MarsRoverMeasures (Autodesk Fusion 360 design; units mm, degrees)
Autodesk Fusion 360 part; units mm, degrees
mesh "Mesh1" [no effect]
ref_plane "WorkPlane2" through (0, 0, 68) normal (0, 0, 1) x (1, 0, 0)
sketch "Top - Wheel" plane through (0, 0, 68) normal (0, 0, 1) x (1, 0, 0)
  line L0 (-376.5767, 66.1614) -> (-266.5767, 66.1614)
  line L1 (-266.5767, 66.1614) -> (-266.5767, -58.8386)
  line L2 (-266.5767, -58.8386) -> (-376.5767, -58.8386)
  line L3 (-376.5767, -58.8386) -> (-376.5767, 66.1614)
  line L4 (293.4233, -58.8386) -> (293.4233, 66.1614)
  line L5 (293.4233, 66.1614) -> (403.4233, 66.1614)
  line L6 (403.4233, 66.1614) -> (403.4233, -58.8386)
  line L7 (403.4233, -58.8386) -> (293.4233, -58.8386)
  line L8 (-376.5767, 3.6614) -> (403.4233, 3.6614) construction
  line L9 (-341.5767, 366.1614) -> (-231.5767, 366.1614)
  line L10 (-231.5767, 366.1614) -> (-231.5767, 241.1614)
  line L11 (-231.5767, 241.1614) -> (-341.5767, 241.1614)
  line L12 (-341.5767, 241.1614) -> (-341.5767, 366.1614)
  line L13 (-341.5767, -393.8386) -> (-341.5767, -268.8386)
  line L14 (-341.5767, -268.8386) -> (-231.5767, -268.8386)
  line L15 (-231.5767, -268.8386) -> (-231.5767, -393.8386)
  line L16 (-231.5767, -393.8386) -> (-341.5767, -393.8386)
  line L17 (258.4233, 241.1614) -> (258.4233, 366.1614)
  line L18 (258.4233, 366.1614) -> (368.4233, 366.1614)
  line L19 (368.4233, 366.1614) -> (368.4233, 241.1614)
  line L20 (368.4233, 241.1614) -> (258.4233, 241.1614)
  line L21 (258.4233, -393.8386) -> (258.4233, -268.8386)
  line L22 (258.4233, -268.8386) -> (368.4233, -268.8386)
  line L23 (368.4233, -393.8386) -> (258.4233, -393.8386)
  line L24 (368.4233, -268.8386) -> (368.4233, -393.8386)
  line L25 (-341.5767, 303.6614) -> (368.4233, 303.6614) construction
  line L26 (-341.5767, -331.3386) -> (368.4233, -331.3386) construction
  line L27 (-266.5767, 66.1614) -> (-266.5767, -58.8386) construction
  line L28 (-231.5767, 241.1614) -> (-231.5767, -268.8386) construction
  line L29 (-321.5767, 66.1614) -> (-321.5767, -58.8386) construction
  line L30 (348.4233, 66.1614) -> (348.4233, -58.8386) construction
  line L31 (-286.5767, 366.1614) -> (-286.5767, 241.1614) construction
  line L32 (313.4233, 366.1614) -> (313.4233, 241.1614) construction
  dimension "d3" = 125
  dimension "d4" = 110
  dimension "d9" = 125
  dimension "d10" = 110
  dimension "d11" = 125
  dimension "d12" = 110
  dimension "d13" = 125
  dimension "d14" = 110
  dimension "d15" = 125
  dimension "d16" = 110
  dimension "d17" = 125
  dimension "d18" = 110
  dimension "d20" = 35
  dimension "d21" = 670
  dimension "d22" = 600
  dimension "d25" = 300
  dimension "d26" = 335
  dimension "d27" = 490
  dimension "d28" = 560
  dimension "d29" = 760
  dimension "d30" = 710
  dimension "d31" = 780
  dimension "d212" = 780
  constraint horizontal L0
  constraint vertical L1
  constraint horizontal L2
  constraint vertical L3
  constraint horizontal L5
  constraint vertical L6
  constraint horizontal L7
  constraint vertical L4
  constraint midpoint L3 L8.start
  constraint midpoint L6 L8.end
  constraint perpendicular L6 L8
  constraint horizontal L9
  constraint vertical L10
  constraint horizontal L11
  constraint vertical L12
  constraint horizontal L14
  constraint vertical L15
  constraint horizontal L16
  constraint vertical L13
  constraint horizontal L18
  constraint vertical L19
  constraint horizontal L20
  constraint vertical L17
  constraint horizontal L22
  constraint vertical L24
  constraint horizontal L23
  constraint vertical L21
  constraint midpoint L12 L25.start
  constraint midpoint L19 L25.end
  constraint perpendicular L19 L25
  constraint midpoint L13 L26.start
  constraint midpoint L24 L26.end
  constraint perpendicular L24 L26
  constraint perpendicular L14 L27
  constraint perpendicular L14 L28
  constraint midpoint L0 L29.start
  constraint perpendicular L2 L29
  constraint midpoint L5 L30.start
  constraint perpendicular L7 L30
  constraint midpoint L9 L31.start
  constraint perpendicular L11 L31
  constraint midpoint L18 L32.start
  constraint perpendicular L20 L32
  constraint midpoint L2 L29.end
  constraint midpoint L7 L30.end
  constraint midpoint L11 L31.end
  constraint midpoint L20 L32.end
  measures "d3" distance of L0.start L2.end
  measures "d4" distance of L0.start L0.end
  measures "d9" distance of L4.start L4.end
  measures "d10" distance of L5.end L4.end
  measures "d11" distance of L9.start L11.end
  measures "d12" distance of L9.start L9.end
  measures "d13" distance of L13.start L13.end
  measures "d14" distance of L14.end L13.end
  measures "d15" distance of L17.start L17.end
  measures "d16" distance of L18.end L17.end
  measures "d17" distance of L21.end L21.start
  measures "d18" distance of L22.end L21.end
  measures "d20" distance of L1.end L28
  measures "d21" distance of L29 L30
  measures "d22" distance of L31 L32
  measures "d25" vertical distance of L8.end L25.end
  measures "d26" vertical distance of L8.end L26.end
  measures "d27" distance of L10.end L17.start
  measures "d28" distance of L1.end L4.start
  measures "d29" distance of L18.end L23.start
  measures "d30" distance of L9.start L18.end
  measures "d31" distance of L0.start L5.end
  measures "d212" distance of L0.start L5.end
ref_plane "WorkPlane3" through (-300, 0, 0) normal (1, 0, 0) x (0, 1, 0)
sketch "Left - Wheel and suspension" plane through (-300, 0, 0) normal (1, 0, 0) x (0, 1, 0)
  line L0 (303.5438, 69.637) -> (-331.4562, 69.637) construction
  circle A0 centre (303.5438, 69.637) radius 62.5
  circle A1 centre (-331.4562, 69.637) radius 62.5
  circle A2 centre (3.5438, 69.637) radius 62.5
  line L1 (-82.4562, 251.637) -> (130.5438, 182.8899)
  line L2 (303.5438, 69.637) -> (303.5438, 201.4155)
  line L3 (303.5438, 201.4155) -> (130.5438, 182.8899)
  line L4 (3.5438, 69.637) -> (3.5438, 107.637)
  line L5 (3.5438, 107.637) -> (130.5438, 182.8899)
  line L6 (-331.4562, 69.637) -> (-331.4562, 193.637)
  line L7 (-331.4562, 193.637) -> (-82.4562, 251.637)
  line L8 (-167.471, 243.4821) -> (-216.657, 232.0251) construction
  line L9 (-213.4962, 209.1456) -> (-162.2533, 221.0817) construction
  line L10 (-167.471, 243.4821) -> (-162.2533, 221.0817) construction
  line L11 (72.0716, 138.0036) -> (92.522, 150.1213) construction
  line L12 (83.8559, 164.7466) -> (59.0651, 150.057) construction
  line L13 (83.8559, 164.7466) -> (92.522, 150.1213) construction
  dimension "d33" = 635
  dimension "d34" = 125
  dimension "d35" = 125
  dimension "d36" = 125
  dimension "d37" = 300
  dimension "d38" = 335
  dimension "d58" = 149
  dimension "d59" = 156
  dimension "d60" = 124
  dimension "d62" = 182
  dimension "d63" = 249
  dimension "d64" = 213
  dimension "d65" = 173
  dimension "d66" = 134.8386
  dimension "d67" = 113.2529
  dimension "d68" = 38
  dimension "d69" = 120.649
  dimension "d70" = 147.6212
  dimension "d71" = 170.1624
  dimension "d400" = 23
  dimension "d401" = 17
  dimension "d454" = 155.464
  dimension "d475" = 103.112
  constraint horizontal L0
  constraint coincident L0.start A0.centre
  constraint coincident L0.end A1.centre
  constraint coincident L0 A2.centre
  constraint perpendicular L0 L2
  constraint coincident A2.centre L4.start
  constraint perpendicular L0 L4
  constraint perpendicular L0 L6
  constraint parallel L7 L9
  constraint perpendicular L9 L10
  constraint perpendicular L8 L10
  constraint parallel L5 L11
  constraint perpendicular L11 L13
  constraint perpendicular L12 L13
  measures "d33" distance of L0.start L0.end
  measures "d34" diameter of A0
  measures "d35" diameter of A1
  measures "d36" diameter of A2
  measures "d37" distance of L0.start A2.centre
  measures "d38" distance of L0.end A2.centre
  measures "d58" angle of L1 L7
  measures "d59" angle of L1 L3
  measures "d60" distance of L0.end L6.end
  measures "d62" vertical distance of L0.end L1.start
  measures "d63" horizontal distance of L1.start L6.end
  measures "d64" horizontal distance of L1.start L1.end
  measures "d65" horizontal distance of L1.end L2.end
  measures "d67" distance of L0 L1.end
  measures "d68" distance of A2.centre L4.end
  measures "d69" angle of L4 L5
  measures "d70" distance of L1.end L4.end
  measures "d71" distance of L1.end A2.centre
  measures "d400" distance of L8.start L9.end
  measures "d401" distance of L11.end L12.start
  measures "d454" angle of L3 L5
  measures "d475" angle of L6 L7
sketch "Left - RTG" plane through (0, 0, 0) normal (1, 0, 0) x (0, 1, 0)
  line L0 (0, 0) -> (0, 467.5219) construction
  line L1 (0, 277.6823) -> (561.1829, 277.6823) construction
  line L2 (210.2843, 277.6823) -> (472.4121, 429.0222) construction
  dimension "d476" = 30
  constraint coincident L0.start origin
  constraint vertical L0
  constraint coincident L0 L1.start
  constraint perpendicular L0 L1
  constraint coincident L1 L2.start
  measures "d476" angle of L1 L2
ref_plane "WorkPlane22" through (12.125, 0, 0) normal (0, 0.866025, 0.5) x (1, 0, 0)
ref_plane "WorkPlane23" through (12.125, 313.5012, 181) normal (0, 0.866025, 0.5) x (1, 0, 0)
ref_plane "WorkPlane4" through (0, 0, 178) normal (0, 0, 1) x (1, 0, 0)
sketch "Top - Wheel and suspension" plane through (0, 0, 178) normal (0, 0, 1) x (1, 0, 0)
  line L0 (-285.6566, 303.5772) -> (-285.6566, -331.4228) construction
  line L1 (-285.6566, 3.5772) -> (-371.3267, 3.5772) construction
  line L2 (-266.7956, 128.5772) -> (-194.7956, 128.5772) construction
  line L3 (-285.6566, 303.5772) -> (-245.2546, 128.5772) construction
  line L4 (-245.2546, 128.5772) -> (-245.2546, -8.4343) construction
  line L5 (-285.6566, -331.4228) -> (-209.2546, -103.3688) construction
  line L6 (-209.2546, -103.3688) -> (-209.2546, 128.5772) construction
  line L7 (-225.0074, -83.4228) -> (-155.0074, -83.4228) construction
  line L8 (-148.5074, 179.005) -> (174.4926, 179.005)
  line L9 (174.4926, 179.005) -> (174.4926, -256.995)
  line L10 (174.4926, -256.995) -> (-148.5074, -256.995)
  line L11 (-148.5074, -256.995) -> (-148.5074, 179.005)
  line L12 (-266.2546, 66.0772) -> (-376.2546, 66.0772)
  line L13 (-376.2546, 66.0772) -> (-376.2546, -58.9228)
  line L14 (-376.2546, -58.9228) -> (-266.2546, -58.9228)
  line L15 (-266.2546, -58.9228) -> (-266.2546, 66.0772)
  line L16 (-199.9544, -33.4769) -> (-199.9544, 51.6617) construction
  line L17 (-221.947, -32.9072) -> (-221.947, 52.0545) construction
  dimension "d73" = 635
  dimension "d74" = 300
  dimension "d75" = 335
  dimension "d76" = 72
  dimension "d77" = 175
  dimension "d78" = 125
  dimension "d79" = 167
  dimension "d80" = 161.478
  dimension "d81" = 70
  dimension "d82" = 87
  dimension "d83" = 248
  dimension "d84" = 436
  dimension "d85" = 323
  dimension "d86" = 6.5
  dimension "d87" = 36
  dimension "d88" = 110
  dimension "d89" = 125
  dimension "d90" = 62.5
  dimension "d91" = 21
  dimension "d211" = 22
  dimension "d473" = 18.522
  dimension "d474" = 13
  constraint vertical L0
  constraint coincident L0 L1.start
  constraint perpendicular L0 L1
  constraint horizontal L2
  constraint coincident L2 L3.end
  constraint perpendicular L2 L4
  constraint coincident L2 L6.end
  constraint perpendicular L2 L6
  constraint perpendicular L6 L7
  constraint horizontal L8
  constraint vertical L9
  constraint horizontal L10
  constraint vertical L11
  constraint horizontal L12
  constraint vertical L13
  constraint horizontal L14
  constraint vertical L15
  constraint perpendicular L2 L16
  constraint vertical L17
  measures "d73" distance of L0.start L0.end
  measures "d74" distance of L0.start L1
  measures "d75" distance of L0.end L1.start
  measures "d76" distance of L2.start L2.end
  measures "d77" vertical distance of L0.start L2.start
  measures "d78" vertical distance of L1.start L2.start
  measures "d79" angle of L3 L4
  measures "d80" angle of L5 L6
  measures "d81" distance of L7.start L7.end
  measures "d82" vertical distance of L1.start L7.start
  measures "d83" vertical distance of L0.end L7.start
  measures "d84" distance of L8.end L9.end
  measures "d85" distance of L9.end L10.end
  measures "d86" distance of L7.end L11
  measures "d87" distance of L3.end L6.end
  measures "d88" distance of L12.start L12.end
  measures "d89" distance of L12.start L14.end
  measures "d90" distance of L1.end L14
  measures "d91" distance of L4.end L15
  measures "d211" distance of L16.start L17.start
  measures "d473" angle of L0 L5
  measures "d474" angle of L0 L3
sketch "Top - Chassis" plane through (0, 0, 178) normal (0, 0, 1) x (1, 0, 0)
  line L0 (311.1042, 304.5371) -> (-284.8958, 304.5371) construction
  line L1 (-284.8958, 304.5371) -> (-284.8958, -330.4629) construction
  line L2 (-284.8958, -330.4629) -> (311.1042, -330.4629) construction
  line L3 (311.1042, -330.4629) -> (311.1042, 304.5371) construction
  line L4 (-266.8958, 64.6219) -> (-376.8958, 64.6219)
  line L5 (-376.8958, 64.6219) -> (-376.8958, -60.3781)
  line L6 (-376.8958, -60.3781) -> (-266.8958, -60.3781)
  line L7 (-266.8958, -60.3781) -> (-266.8958, 64.6219)
  line L8 (403.1042, -60.3781) -> (403.1042, 64.6219)
  line L9 (403.1042, 64.6219) -> (293.1042, 64.6219)
  line L10 (293.1042, 64.6219) -> (293.1042, -60.3781)
  line L11 (293.1042, -60.3781) -> (403.1042, -60.3781)
  line L12 (174.6042, 178.5371) -> (-148.3958, 178.5371)
  line L13 (-148.3958, 178.5371) -> (-148.3958, -256.4629)
  line L14 (-148.3958, -256.4629) -> (174.6042, -256.4629)
  line L15 (174.6042, -256.4629) -> (174.6042, 178.5371)
  line L16 (-341.6412, 372.3911) -> (368.3588, 372.3911) construction
  line L17 (-341.6412, -397.6089) -> (368.3588, -397.6089) construction
  line L18 (-341.6412, 372.3911) -> (-341.6412, -397.6089) construction
  line L19 (368.3588, 372.3911) -> (368.3588, -397.6089) construction
  line L20 (174.6042, -38.9629) -> (-148.3958, -38.9629) construction
  line L21 (174.6042, 17.0371) -> (-148.3958, 17.0371) construction
  line L22 (-148.3958, -87.6567) -> (-165.872, -87.6567)
  dimension "d93" = 635
  dimension "d94" = 596
  dimension "d95" = 110
  dimension "d96" = 125
  dimension "d97" = 110
  dimension "d98" = 125
  dimension "d99" = 18
  dimension "d100" = 18
  dimension "d101" = 780
  dimension "d102" = 323
  dimension "d103" = 435
  dimension "d106" = 136.5
  dimension "d107" = 136.5
  dimension "d109" = 126
  dimension "d110" = 74
  dimension "d241" = 710
  dimension "d402" = 770
  dimension "d455" = 56
  constraint horizontal L0
  constraint vertical L1
  constraint horizontal L2
  constraint vertical L3
  constraint horizontal L4
  constraint vertical L5
  constraint horizontal L6
  constraint vertical L7
  constraint horizontal L9
  constraint vertical L10
  constraint horizontal L11
  constraint vertical L8
  constraint horizontal L12
  constraint vertical L13
  constraint horizontal L14
  constraint vertical L15
  constraint horizontal L17
  constraint coincident L17 L18.end
  constraint coincident L17 L19.end
  constraint midpoint L15 L20.start
  constraint midpoint L13 L20.end
  constraint coincident L15 L21.start
  constraint coincident L13 L21.end
  constraint perpendicular L13 L21
  constraint coincident L13 L22.start
  constraint perpendicular L13 L22
  measures "d93" distance of L0.start L2.end
  measures "d94" distance of L0.start L0.end
  measures "d95" distance of L4.start L4.end
  measures "d96" distance of L4.start L6.end
  measures "d97" distance of L9.end L8.end
  measures "d98" distance of L8.start L8.end
  measures "d99" distance of L1 L6.end
  measures "d100" distance of L3 L10.end
  measures "d101" distance of L4.end L8.end
  measures "d102" distance of L12.start L12.end
  measures "d103" distance of L12.start L14.end
  measures "d106" horizontal distance of L2.end L14.end
  measures "d107" horizontal distance of L1.end L13.end
  measures "d109" vertical distance of L0.start L12.start
  measures "d110" vertical distance of L2.end L14.end
  measures "d241" distance of L16.start L16.end
  measures "d402" distance of L16.start L17.start
  measures "d455" distance of L20 L21
ref_plane "WorkPlane5" through (0, -225, 0) normal (0, 1, 0) x (0, 0, 1)
sketch "Front - Chassis and Cam" plane through (0, -225, 0) normal (0, 1, 0) x (1, 0, 0)
  line L0 (-148.2843, -313) -> (174.7157, -313)
  line L1 (174.7157, -313) -> (174.7157, -185)
  line L2 (174.7157, -185) -> (-148.2843, -185)
  line L3 (-148.2843, -185) -> (-148.2843, -313)
  line L4 (-53.8892, -564) -> (-202.3892, -564)
  line L5 (-202.3892, -564) -> (-202.3892, -571)
  line L6 (-202.3892, -571) -> (-53.8892, -571)
  line L7 (-53.8892, -571) -> (-53.8892, -564)
  line L8 (-196.9099, -614) -> (-70.9099, -614)
  line L9 (-70.9099, -614) -> (-70.9099, -571)
  line L10 (-70.9099, -571) -> (-196.9099, -571)
  line L11 (-196.9099, -571) -> (-196.9099, -614)
  line L12 (-189.3792, -621) -> (-77.8792, -621)
  line L13 (-70.9099, -571) -> (-60.6099, -571)
  line L14 (-60.6099, -571) -> (-60.6099, -585.7)
  line L15 (-60.6099, -585.7) -> (-70.9099, -585.7)
  line L16 (-70.9099, -585.7) -> (-70.9099, -571)
  line L17 (-158.5751, -506.4898) -> (-128.2751, -506.4898)
  line L18 (-128.2751, -506.4898) -> (-128.2751, -485.8898)
  line L19 (-128.2751, -485.8898) -> (-158.5751, -485.8898)
  line L20 (-158.5751, -485.8898) -> (-158.5751, -506.4898)
  dimension "d112" = 323
  dimension "d113" = 128
  dimension "d114" = 148.5
  dimension "d115" = 7
  dimension "d116" = 43
  dimension "d117" = 126
  dimension "d118" = 111.5
  dimension "d119" = 7
  dimension "d120" = 251
  dimension "d124" = 14.7
  dimension "d125" = 10.3
  dimension "d213" = 30.3
  dimension "d215" = 20.6
  dimension "d388" = 571
  constraint horizontal L0
  constraint vertical L1
  constraint horizontal L2
  constraint vertical L3
  constraint horizontal L4
  constraint vertical L5
  constraint horizontal L6
  constraint vertical L7
  constraint horizontal L8
  constraint vertical L9
  constraint horizontal L10
  constraint vertical L11
  constraint coincident L6 L9.end
  constraint horizontal L12
  constraint horizontal L13
  constraint vertical L14
  constraint horizontal L15
  constraint vertical L16
  constraint horizontal L17
  constraint vertical L18
  constraint horizontal L19
  constraint vertical L20
  measures "d112" distance of L0.start L0.end
  measures "d113" distance of L0.end L1.end
  measures "d114" distance of L5 L7
  measures "d115" distance of L4.end L5.end
  measures "d116" distance of L8.start L10.end
  measures "d117" distance of L8.start L8.end
  measures "d118" distance of L12.start L12.end
  measures "d119" vertical distance of L8.end L12.end
  measures "d120" distance of L0.start L4
  measures "d124" distance of L13.end L14.end
  measures "d125" distance of L14.end L15.end
  measures "d213" distance of L18.end L19.end
  measures "d215" distance of L17.start L19.end
  measures "d388" vertical distance of origin L9.end
ref_plane "WorkPlane10" through (-386.1613, -337.5, 781.806) normal (0, 0, 1) x (1, 0, 0)
sketch "Sketch19" plane through (0, 0, 781.806) normal (0, 0, 1) x (-1, 0, 0)
  circle A0 centre (142.453, 225.0109) radius 33
  circle A1 centre (143.6218, 222.8237) radius 15
  dimension "d392" = 30
  measures "d392" diameter of A1
ref_plane "WorkPlane11" through (0, -220, 0) normal (0, 1, 0) x (0, 0, 1)
sketch "Sketch20" plane through (0, -220, 0) normal (0, 1, 0) x (1, 0, 0)
  line L0 (-158.6064, -506.0999) -> (-128.6064, -506.0999)
  line L1 (-128.6064, -506.0999) -> (-128.6064, -486.0999)
  line L2 (-128.6064, -486.0999) -> (-158.6064, -486.0999)
  line L3 (-158.6064, -486.0999) -> (-158.6064, -506.0999)
  line L4 (-128.6064, -486.0999) -> (-158.6064, -486.0999)
  line L5 (-200.2466, -474.0999) -> (-113.4124, -474.0999) construction
  line L6 (-201.8884, -563.5999) -> (-61.2389, -563.5999) construction
  line L7 (-181.6393, -535.0999) -> (-87.5081, -535.0999) construction
  dimension "d394" = 20
  dimension "d395" = 30
  dimension "d396" = 12
  dimension "d397" = 28.5
  dimension "d398" = 29
  dimension "d399" = 89.7
  constraint horizontal L0
  constraint vertical L1
  constraint horizontal L2
  constraint vertical L3
  constraint horizontal L4
  constraint horizontal L5
  constraint horizontal L6
  constraint parallel L6 L7
  measures "d394" distance of L0.start L2.end
  measures "d395" distance of L0.start L0.end
  measures "d396" distance of L2 L5
  measures "d397" distance of L6 L7
  measures "d398" distance of L0 L7
extrude "Extrude20" add sketch "Sketch19" along normal blind 21 contours A1
ref_plane "WorkPlane12" through (0, -260, 0) normal (0, 1, 0) x (0, 0, 1)
sketch "Sketch21" plane through (0, -260, 0) normal (0, 1, 0) x (1, 0, 0)
  circle A0 centre (-190.1986, -557.4012) radius 4.5
  line L0 (-183.1986, -551.9012) -> (-197.1986, -551.9012)
  line L1 (-197.1986, -551.9012) -> (-197.1986, -562.9012)
  line L2 (-197.1986, -562.9012) -> (-183.1986, -562.9012)
  line L3 (-183.1986, -562.9012) -> (-183.1986, -551.9012)
  line L4 (-183.1986, -551.9012) -> (-197.1986, -562.9012) construction
  line L5 (-197.1986, -551.9012) -> (-183.1986, -562.9012) construction
  point P0 (-190.1986, -557.4012)
  dimension "d403" = 9
  dimension "d405" = 11
  dimension "d406" = 14
  constraint perpendicular L0 L1
  constraint parallel L0 L2
  constraint parallel L1 L3
  constraint horizontal L0
  constraint coincident L4 P0
  constraint coincident L5 P0
  constraint coincident P0 A0.centre
  measures "d403" diameter of A0
  measures "d405" distance of L0.start L2.end
  measures "d406" distance of L0.start L0.end
sketch "Sketch24" plane through (0, 0, 310.1429) normal (0, 0, 1) x (-1, 0, 0)
  line L0 (154.6751, 110.682) -> (148.6751, 121.682)
  line L1 (148.6751, 121.682) -> (147.6751, 121.682)
  line L2 (147.6751, 121.682) -> (147.6751, 55.682)
  line L3 (147.6751, 55.682) -> (154.6751, 55.682)
  line L4 (154.6751, 55.682) -> (154.6751, 110.682)
ref_plane "WorkPlane13" through (0, 0, 250) normal (0, 0, 1) x (1, 0, 0)
sketch "Sketch25" plane through (0, 0, 250) normal (0, 0, 1) x (1, 0, 0)
ref_plane "WorkPlane14" through (192.3249, -83.182, 249.1429) normal (1, 0, 0) x (0, -1, 0)
sketch "Sketch27" plane through (192.3249, -83.182, 249.1429) normal (1, 0, 0) x (0, 1, 0)
  line L0 (88.1106, 71.7156) -> (-35.2917, 71.7156) construction
  circle A0 centre (0.3753, -3.4844) radius 19.5
  line L1 (0.3753, -3.4844) -> (0.3753, 71.7156) construction
  line L2 (-19.1247, -3.4844) -> (19.8753, -3.4844) construction
  line L3 (-3.4747, 71.7156) -> (-17.6247, -3.4844)
  circle A1 centre (0.3753, -3.4844) radius 18
  circle A2 centre (0.3753, 71.7156) radius 3.85
  dimension "d418" = 39
  dimension "d420" = 36
  dimension "d421" = 7.7
  dimension "d422" = 75.2
  constraint horizontal L0
  constraint coincident A0.centre L1.start
  constraint coincident L0 L1.end
  constraint perpendicular L0 L1
  constraint coincident A0 L2.start
  constraint coincident A0 L2.end
  constraint coincident A0.centre L2
  constraint horizontal L2
  constraint coincident L2 L3.end
  constraint coincident L3.end A1
  constraint coincident L0 L3.start
  constraint coincident L1.end A2.centre
  constraint coincident L3.start A2
  measures "d418" diameter of A0
  measures "d420" diameter of A1
  measures "d421" diameter of A2
  measures "d422" distance of A0.centre L1.end
sketch "Sketch28" plane through (0, 0, 250) normal (0, 0, 1) x (1, 0, 0)
sketch "Sketch29" plane through (0, 0, 250) normal (0, 0, 1) x (1, 0, 0)
sketch "Sketch30" plane through (0, 0, 250) normal (0, 0, 1) x (1, 0, 0)
ref_plane "WorkPlane15" through (0, -80, 0) normal (0, 1, 0) x (0, 0, 1)
sketch "Sketch31" plane through (0, -80, 0) normal (0, 1, 0) x (1, 0, 0)
  line L0 (-218.1313, -260.6757) -> (-224.4446, -230.974)
  line L1 (-214.1751, -224.3429) -> (-214.1751, -267.3429)
  line L2 (-219.1751, -265.3429) -> (-219.1751, -226.3429)
  line L3 (-219.1751, -245.8429) -> (-221.288, -245.8429)
  line L4 (-221.288, -245.8429) -> (-221.288, -245.8249)
  line L5 (-221.288, -245.8249) -> (-219.1751, -245.8249)
  line L6 (-219.1751, -245.8249) -> (-219.1751, -245.8429)
  line L7 (-216.1751, -260.2599) -> (-222.4883, -230.5582)
  line L8 (-219.1751, -260.5202) -> (-219.1751, -230)
  line L9 (-219.1751, -245.8429) -> (-219.1751, -260.3429)
  line L10 (-219.1751, -245.8429) -> (-219.1751, -231.3429)
  line L11 (-249.7499, -267.3964) -> (-256.0631, -237.6947)
  dimension "d424" = 2
  dimension "d427" = 12
  dimension "d428" = 14.5
  dimension "d429" = 14.5
  dimension "d430" = 3
  dimension "d431" = -32.3249
  constraint horizontal L3
  constraint vertical L4
  constraint horizontal L5
  constraint vertical L6
  constraint midpoint L0 L4.end
  constraint midpoint L2 L3.start
  constraint coincident L2 L8.start
  constraint perpendicular L3 L8
  constraint perpendicular L5 L9
  constraint perpendicular L5 L10
  measures "d427" angle of L7 L8
  measures "d428" distance of L3.start L9.end
  measures "d429" distance of L3.start L10.end
  measures "d430" distance of L7.start L8
ref_plane "WorkPlane16" through (-239.4269, -82.182, 248.833) normal (0.198827, -0.292372, 0.935407) x (-0.978148, 0, 0.207912)
sketch "Sketch32" plane through (-210.6129, -80.4381, 243.2534) normal (0.198827, -0.292372, 0.935407) x (-0.978148, 0, 0.207912)
  line L0 (39.7719, 116.5078) -> (31.2227, 82.2187)
  line L1 (17.4551, 122.072) -> (8.9059, 87.7829)
  line L2 (5, 0) -> (26.9699, 0)
  line L3 (18.6443, 21.3232) -> (-8.8557, 21.3232)
  line L4 (-8.8557, 21.3232) -> (-8.8557, -17.5495)
  line L5 (-8.8557, -17.5495) -> (18.6443, -17.5495)
  line L6 (18.6443, -17.5495) -> (18.6443, 21.3232)
  dimension "d433" = 23
  dimension "d435" = 76
  dimension "d436" = 27.5
  dimension "d437" = 14
  constraint horizontal L2
  constraint horizontal L3
  constraint vertical L4
  constraint horizontal L5
  constraint vertical L6
  measures "d435" angle of L0 L2
  measures "d436" distance of L3.start L3.end
  measures "d437" angle of L1 L4
ref_plane "WorkPlane17" through (0, 0, 320) normal (0, 0, 1) x (1, 0, 0)
sketch "Sketch33" plane through (0, 0, 320) normal (0, 0, 1) x (1, 0, 0)
  line L0 (-167.1178, 16.9441) -> (191.8822, 16.9441) construction
  circle A0 centre (-167.1178, 16.9441) radius 3
  circle A1 centre (191.8822, 16.9441) radius 3
  circle A2 centre (12.3822, 16.9441) radius 12.5
  circle A3 centre (12.3822, 16.9441) radius 18.5
  circle A4 centre (-167.1178, 16.9441) radius 6.25
  circle A5 centre (191.8822, 16.9441) radius 6.25
  line L1 (12.3822, 36.9441) -> (12.3822, -3.0559) construction
  line L2 (-9.2181, -3.0559) -> (33.9826, -3.0559)
  line L3 (-20.1178, 36.9441) -> (44.8822, 36.9441)
  line L4 (-20.1178, 36.9441) -> (-167.6987, 23.167)
  line L5 (-9.2181, -3.0559) -> (-167.6591, 10.7176)
  line L6 (33.9826, -3.0559) -> (192.4235, 10.7176)
  line L7 (44.8822, 36.9441) -> (192.4631, 23.167)
  dimension "d439" = 359
  dimension "d440" = 6
  dimension "d441" = 6
  dimension "d442" = 25
  dimension "d443" = 37
  dimension "d444" = 12.5
  dimension "d445" = 12.5
  dimension "d446" = 20
  dimension "d447" = 65
  dimension "d448" = 20
  constraint horizontal L0
  constraint coincident L0.start A0.centre
  constraint coincident L0.end A1.centre
  constraint midpoint L0 A2.centre
  constraint concentric A2 A3
  constraint concentric A0 A4
  constraint concentric A1 A5
  constraint perpendicular L0 L1
  constraint perpendicular L1 L3
  constraint midpoint L1.start L3
  constraint midpoint L1.end L2
  constraint horizontal L2
  constraint midpoint A2.centre L1
  constraint coincident A4 L4.end
  constraint tangent A4 L4
  constraint coincident A4 L5.end
  constraint tangent A4 L5
  constraint coincident A5 L6.end
  constraint tangent A5 L6
  constraint coincident A5 L7.end
  constraint tangent A5 L7
  measures "d439" distance of L0.start L0.end
  measures "d440" diameter of A0
  measures "d441" diameter of A1
  measures "d442" diameter of A2
  measures "d443" diameter of A3
  measures "d444" diameter of A4
  measures "d445" diameter of A5
  measures "d446" distance of A2.centre L1.end
  measures "d447" distance of L3.start L3.end
  measures "d448" vertical distance of A2.centre L1.start
ref_plane "WorkPlane18" through (0, 0, 180) normal (0, 0, 1) x (1, 0, 0)
sketch "Sketch34" plane through (0, 0, 180) normal (0, 0, 1) x (1, 0, 0)
  line L0 (-227.4262, 140.0762) -> (-260.9262, 140.0762)
  line L1 (-260.9262, 140.0762) -> (-260.9262, 117.0762)
  line L2 (-260.9262, 117.0762) -> (-227.4262, 117.0762)
  line L3 (-227.4262, 117.0762) -> (-227.4262, 140.0762)
  line L4 (-194.9262, 145.571) -> (-227.4262, 145.571)
  line L5 (-227.4262, 145.571) -> (-227.4262, 112.071)
  line L6 (-227.4262, 112.071) -> (-194.9262, 112.071)
  line L7 (-194.9262, 112.071) -> (-194.9262, 145.571)
  dimension "d450" = 33.5
  dimension "d451" = 32.5
  dimension "d452" = 23
  dimension "d453" = 33.5
  constraint horizontal L0
  constraint vertical L1
  constraint horizontal L2
  constraint vertical L3
  constraint horizontal L4
  constraint vertical L5
  constraint horizontal L6
  constraint vertical L7
  constraint coincident L2.end L5
  measures "d450" distance of L4.start L6.end
  measures "d451" distance of L4.start L4.end
  measures "d452" distance of L0.start L2.end
  measures "d453" distance of L1.end L2.end
ref_plane "WorkPlane20" through (0, 180, 0) normal (0, 1, 0) x (0, 0, 1)
sketch "Sketch44" plane through (0, 180, 0) normal (0, 1, 0) x (1, 0, 0)
  line L0 (175.3135, -188.3884) -> (130.3135, -188.3884)
  line L1 (130.3135, -188.3884) -> (130.3135, -310.1884)
  line L2 (130.3135, -310.1884) -> (175.3135, -310.1884)
  line L3 (175.3135, -310.1884) -> (175.3135, -188.3884)
  dimension "d493" = 45
  dimension "d494" = 121.8
  constraint horizontal L0
  constraint vertical L1
  constraint horizontal L2
  constraint vertical L3
  measures "d493" distance of L0.start L0.end
  measures "d494" distance of L0.end L1.end
sketch "Sketch45" plane through (192.3249, -83.182, 249.1429) normal (1, 0, 0) x (0, 1, 0)
  line L0 (262.5517, 63.7544) -> (262.5517, -58.0456)
  line L1 (344.5517, 118.0898) -> (344.5517, -36.0738)
  line L2 (262.5517, 63.7544) -> (306.5517, 118.0898)
  line L3 (306.5517, 118.0898) -> (344.5517, 118.0898)
  line L4 (344.5517, -36.0738) -> (262.5517, -58.0456)
  dimension "d495" = 121.8
  dimension "d496" = 82
  dimension "d497" = 38
  dimension "d498" = 141
  dimension "d499" = 75
  constraint vertical L0
  constraint vertical L1
  constraint perpendicular L1 L3
  measures "d495" distance of L0.start L0.end
  measures "d496" distance of L0 L1
  measures "d497" distance of L1.start L2.end
  measures "d498" angle of L0 L2
  measures "d499" angle of L0 L4
hidden bodies 1
equation "Trous_Vis_diam2 = 2.2 mm"
